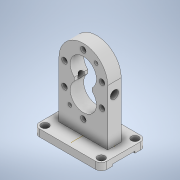
# Autodesk Inventor part: Součást2
Saved by Autodesk Inventor 2022 (Build 260153000, 153)
## iProperties
Created: 2022-04-03
Part Number: Součást2
Material: Všeobecné
Document SubType Name: Modeling
Designer: Šimon
Density: 1 g/cm^3
Appearance: Výchozí
Author: Šimon
Autodesk Inventor part; units mm, degrees
note: some values were not read from the file. Chosen so that the rebuilt part matches the saved one: pattern direction of "Obdélníkové pole1".
ref_plane "YZ Plane" through (0, 0, 0) normal (1, 0, 0) x (0, 1, 0)
ref_plane "XZ Plane" through (0, 0, 0) normal (0, 1, 0) x (-1, 0, 0)
ref_plane "XY Plane" through (0, 0, 0) normal (0, 0, 1) x (1, 0, 0)
sketch "Náčrt1" plane through (0, 0, 0) normal (0, 1, 0) x (-1, 0, 0)
  line L0 (-15.3978, 30.8958) -> (-135.3978, 30.8958)
  line L1 (-165.3978, 0.8958) -> (-165.3978, -63.1461)
  line L2 (-135.6713, -89.1042) -> (-15.3978, -89.1042)
  line L3 (14.6022, -59.1042) -> (14.6022, 0.8958)
  line L4 (-15.3978, -89.1042) -> (14.6022, -89.1042)
  line L5 (14.6022, -89.1042) -> (14.6022, -59.1042)
  line L6 (14.6022, 0.8958) -> (14.6022, 30.8958)
  line L7 (14.6022, 30.8958) -> (-15.3978, 30.8958)
  line L8 (-135.3978, 30.8958) -> (-165.3978, 30.8958)
  line L9 (-165.3978, 30.8958) -> (-165.3978, 0.8958)
  line L10 (-165.3978, -63.1461) -> (-165.3978, -89.1042)
  line L11 (-135.6713, -89.1042) -> (-165.3978, -89.1042)
  point P0 (0, 0)
  dimension "d4" = 180
  dimension "d5" = 120
  constraints: 24 end point, 6 perpendicular, 4 point on line, 2 horizontal, 1 vertical
  measures "d4" distance between parallel lines of L3 L1
  measures "d5" distance between parallel lines of L0 L2
extrude "Vysunutí1" add sketch "Náčrt1" along normal blind 19
ref_plane "Pracovní rovina1" through (15.3978, 0, -29.1042) normal (0, 0, 1) x (1, 0, 0)
sketch "Náčrt2" plane through (15.3978, 0, -29.1042) normal (0, 0, 1) x (1, 0, 0)
  line L0 (0, 19) -> (-30, 19) projected
  line L1 (150, 19) -> (-30, 19) projected
  line L2 (-4.8632, 19) -> (-4.8632, 168)
  arc A0 (125.1368, 168) -> (-4.8632, 168) centre (60.1368, 168) ccw
  line L3 (125.1368, 168) -> (125.1368, 19)
  line L4 (-4.8632, 19) -> (125.1368, 19)
  line L5 (150, 0) -> (-30, 0) projected
  line L6 (36.1368, 133.4755) -> (36.1368, 142.5245)
  line L7 (84.1368, 142.5245) -> (84.1368, 133.4755)
  arc A1 (36.1368, 133.4755) -> (84.1368, 133.4755) centre (60.1368, 108) ccw
  arc A2 (84.1368, 142.5245) -> (36.1368, 142.5245) centre (60.1368, 168) ccw
  point P0 (-15.3978, 0)
  point P1 (120.2735, 19)
  point P2 (60.1368, 0)
  point P3 (120.2735, 0)
  point P4 (0, 0)
  point P5 (120.2735, 19)
  dimension "d10" = 130
  dimension "d11" = 168
  dimension "d15" = 60
  dimension "d16" = 24
  dimension "d17" = 24
  constraints: 10 end point, 6 point on circle, 3 centre point, 3 point on line, 3 vertical, 2 tangent, 1 coincident, 1 parallel, 1 perpendicular, 1 vertical alignment
  measures "d10" distance between parallel lines of L2 L3
  measures "d11" distance of point (60.137, 0) A0.centre
  measures "d15" distance of A1.centre A0.centre
  measures "d16" distance from line of A1.centre L6
  measures "d17" distance from line of L7 A1.centre
extrude "Vysunutí2" add sketch "Náčrt2" along normal mid plane 36
sketch "Náčrt3" plane through (15.3978, 0, -29.1042) normal (0, 0, 1) x (1, 0, 0)
  line L0 (166.8566, 138) -> (-66.006, 138)
  line L1 (-9.4318, 138) -> (-9.4318, 149)
  line L2 (-9.4318, 149) -> (14.2974, 149)
  line L3 (14.2974, 149) -> (14.2974, 147)
  line L4 (14.2974, 147) -> (88.3325, 147)
  line L5 (88.3325, 147) -> (109.5306, 147)
  line L6 (109.5306, 147) -> (109.5306, 149)
  line L7 (109.5306, 149) -> (145.9153, 149)
  line L8 (145.9153, 149) -> (145.9153, 138)
  line L9 (-9.4318, 138) -> (145.9153, 138)
  line L10 (36.1368, 142.5245) -> (36.1368, 133.4755) projected
  point P0 (-15.3978, 0)
  point P1 (36.1368, 138)
  dimension "d20" = 22
  dimension "d21" = 18
  dimension "d22" = 0
  constraints: 20 end point, 5 perpendicular, 5 point on line, 1 horizontal, 1 midpoint
  measures "d20" diameter of L7 L0
  measures "d21" diameter of L4 L0
  measures "d22" distance from line of point (36.137, 138) L0
revolve "Rotace1" cut sketch "Náčrt3" angle 360 about axis through (182.2543, 138, -29.1042) along (-1, 0, 0)
sketch "Náčrt6" plane through (0, 19, 0) normal (0, 1, 0) x (1, 0, 0)
  line L0 (-14.6022, 89.1042) -> (-14.6022, -30.8958) projected
  line L1 (-14.6022, -30.8958) -> (165.3978, -30.8958) projected
  point P0 (0, 0)
  point P1 (0.3978, -15.8958)
  point P2 (-14.6022, 59.1042)
  point P3 (-14.6022, -0.8958)
  point P4 (15.3978, -30.8958)
  point P5 (135.3978, -30.8958)
  dimension "d34" = 15
  dimension "d35" = 15
  measures "d34" distance from line of L0 point (0.398, -15.896)
  measures "d35" distance from line of L1 point (0.398, -15.896)
hole "Díra1" at (0.3978, 19, 15.8958) direction (0, -1, 0) diameter 15 end through all counterbore diameter 20 counterbore depth 13
sketch "Náčrt7" plane through (0, 19, 0) normal (0, 1, 0) x (1, 0, 0)
  line L0 (150.5345, -15.8958) -> (0.5345, -15.8958)
  line L1 (0.5345, -15.8958) -> (0.5345, 74.1042)
  line L2 (0.5345, 74.1042) -> (150.5345, 74.1042)
  line L3 (150.5345, 74.1042) -> (150.5345, -15.8958)
  line L4 (165.3978, 89.1042) -> (-14.6022, 89.1042) projected
  line L5 (-14.6022, 89.1042) -> (-14.6022, -30.8958) projected
  point P0 (0, 0)
  point P1 (75.5345, 74.1042)
  point P2 (75.5345, 89.1042)
  point P3 (135.6713, 89.1042)
  point P4 (15.3978, 89.1042)
  point P5 (0.5345, 29.1042)
  point P6 (-14.6022, 29.1042)
  point P7 (-14.6022, 59.1042)
  point P8 (-14.6022, -0.8958)
  dimension "d32" = 90
  dimension "d33" = 150
  constraints: 8 end point, 3 midpoint, 2 parallel, 1 horizontal, 1 horizontal alignment, 1 perpendicular, 1 point on line, 1 vertical alignment
  measures "d32" distance between parallel lines of L0 L2
  measures "d33" distance between parallel lines of L3 L1
fillet "Zaoblení1" radius 15 4 edges at (-14.6022, 9.5, 30.8958) (165.3978, 9.5, 30.8958) (165.3978, 9.5, -89.1042) (-14.6022, 9.5, -89.1042)
pattern_linear "Obdélníkové pole1" count 2 spacing -150 along (-1, 0, 0) count 2 spacing 90 along (0, 0, -1) of "Díra1"
sketch "Náčrt8" plane through (15.3978, 0, -11.1042) normal (0, 0, 1) x (1, 0, 0)
  arc A0 (84.1368, 142.5245) -> (36.1368, 142.5245) centre (60.1368, 168) ccw projected
  arc A1 (100.1368, 138) -> (20.1368, 138) centre (60.1368, 168) ccw
  arc A2 (36.1368, 133.4755) -> (84.1368, 133.4755) centre (60.1368, 108) ccw projected
  arc A3 (20.1368, 138) -> (100.1368, 138) centre (60.1368, 108) ccw
  point P0 (-15.3978, 0)
  point P1 (110.1368, 168)
  point P2 (10.1368, 168)
  point P3 (60.1368, 58)
  point P4 (110.1368, 108)
  point P5 (10.1368, 108)
  dimension "d43" = 100
  dimension "d44" = 100
  constraints: 9 point on circle, 2 centre point, 2 coincident
  measures "d43" diameter of A1
  measures "d44" diameter of A3
ref_plane "Pracovní rovina2" through (75.3978, 0, 15.8958) normal (1, 0, 0) x (0, 0, -1)
sketch "Náčrt9" plane through (75.3978, 0, 15.8958) normal (1, 0, 0) x (0, 0, -1)
  line L0 (15.8958, 218) -> (92.8, 218)
  line L1 (27, 233) -> (27, 168) projected
  line L2 (27, 218) -> (27, 225.5)
  line L3 (27, 225.5) -> (35, 225.5)
  line L4 (35, 225.5) -> (35, 224)
  line L5 (35, 224) -> (55, 224)
  line L6 (55, 224) -> (55, 225.5)
  line L7 (55, 225.5) -> (63, 225.5)
  line L8 (63, 168) -> (63, 233) projected
  line L9 (63, 218) -> (63, 225.5)
  line L10 (27, 218) -> (63, 218)
  line L11 (0, 0) -> (-15, 0) projected
  point P0 (15.8958, 0)
  dimension "d46" = 15
  dimension "d47" = 12
  dimension "d48" = 8
  dimension "d49" = 8
  dimension "d53" = 15
  constraints: 18 end point, 8 point on line, 3 perpendicular, 2 collinear, 2 horizontal
  measures "d46" diameter of L7 L0
  measures "d47" diameter of L5 L0
  measures "d48" distance between parallel lines of L1 L4
  measures "d49" distance between parallel lines of L8 L6
  measures "d53" distance of L1.start L2.start
revolve "Rotace2" cut sketch "Náčrt9" angle 360 about axis through (75.3978, 218, 0) along (0, 0, -1)
pattern_sketch "Pole řízené náčrtem1" of "Rotace2" from (75.3978, 218, -11.1042) copies at (125.5345, 168, -11.1042) at (25.5345, 168, -11.1042) at (75.5345, 58, -11.1042) at (125.5345, 108, -11.1042) at (25.5345, 108, -11.1042)
sketch "Náčrt10" plane through (15.3978, 0, -11.1042) normal (0, 0, 1) x (1, 0, 0)
  arc A0 (84.1368, 142.5245) -> (36.1368, 142.5245) centre (60.1368, 168) ccw projected
  circle A1 centre (10.1368, 168) radius 6 projected
  circle A2 centre (60.1368, 168) radius 50
  arc A3 (36.1368, 133.4755) -> (84.1368, 133.4755) centre (60.1368, 108) ccw projected
  circle A4 centre (60.1368, 58) radius 6 projected
  circle A5 centre (60.1368, 108) radius 50
  circle A6 centre (24.4365, 72.993) radius 5
  circle A7 centre (94.5409, 204.2816) radius 5
  point P0 (-15.3978, 0)
  dimension "d54" = 10
  dimension "d55" = 10
  constraints: 4 centre point, 4 point on circle, 2 coincident
  measures "d54" diameter of A6
  measures "d55" diameter of A7
extrude "Vysunutí3" cut sketch "Náčrt10" against normal through all contours A6 A5 | A5 A6 | A7 A2 | A2 A7
sketch "Náčrt11" plane through (165.3978, 0, 15.8958) normal (1, 0, 0) x (0, 0, -1)
  line L0 (0, 0) -> (90, 0) projected
  line L1 (15, 5) -> (75, 5)
  line L2 (75, 5) -> (75, 0)
  line L3 (75, 0) -> (15, 0)
  line L4 (15, 0) -> (15, 5)
  line L5 (0, 19) -> (90, 19) projected
  point P0 (45, 5)
  point P1 (45, 19)
  point P2 (15, 0)
  dimension "d61" = 60
  dimension "d62" = 5
  constraints: 8 end point, 2 midpoint, 2 parallel, 1 horizontal, 1 perpendicular, 1 point on line, 1 vertical alignment
  measures "d61" distance between parallel lines of L2 L4
  measures "d62" distance between parallel lines of L0 L1
extrude "Vysunutí4" cut sketch "Náčrt11" against normal through all
